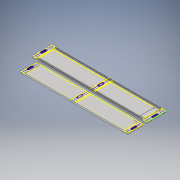
# Autodesk Inventor part: Fixture Base
Saved by Autodesk Inventor 2018 (Build 220112000, 112)
## iProperties
Created: 2016-04-07
Part Number: Fixture Base
Material: Generic
Document SubType Name: Modeling
Designer: Sam Clay
Density: 1 g/cm^3
Appearance: Default
Author: Sam Clay
Autodesk Inventor part; units mm, degrees
ref_plane "YZ Plane" through (0, 0, 0) normal (1, 0, 0) x (0, 1, 0)
ref_plane "XZ Plane" through (0, 0, 0) normal (0, 1, 0) x (-1, 0, 0)
ref_plane "XY Plane" through (0, 0, 0) normal (0, 0, 1) x (1, 0, 0)
sketch "Base Sketch" plane through (0, 0, 0) normal (0, 1, 0) x (-1, 0, 0)
  line L0 (0, 0) -> (1422.4, 0)
  line L1 (1422.4, 0) -> (1422.4, 254)
  line L2 (1320.8, 508) -> (0, 508)
  line L3 (0, 508) -> (0, 304.8)
  line L4 (0, 508) -> (-50.8, 508)
  line L5 (-50.8, 508) -> (-50.8, 304.8)
  line L6 (-50.8, 0) -> (0, 0)
  line L7 (0, 0) -> (0, 254)
  line L8 (1320.8, 508) -> (1371.6, 508)
  line L9 (1371.6, 508) -> (1371.6, 304.8)
  line L10 (1473.2, 0) -> (1422.4, 0)
  line L11 (1422.4, 0) -> (1422.4, 254)
  line L12 (1473.2, 254) -> (1473.2, 0)
  line L13 (0, 254) -> (0, 254)
  line L14 (-50.8, 223.384) -> (-50.8, 0)
  line L15 (1371.6, 304.8) -> (1320.8, 304.8)
  line L16 (1320.8, 304.8) -> (1320.8, 508)
  line L17 (-50.8, 254) -> (-50.8, 223.384)
  line L18 (1422.4, 254) -> (0, 254)
  line L19 (1320.8, 304.8) -> (0, 304.8)
  line L20 (0, 304.8) -> (-50.8, 304.8)
  line L21 (0, 254) -> (-50.8, 254)
  line L22 (0, 304.8) -> (0, 508)
  line L23 (0, 254) -> (0, 0)
  line L24 (1320.8, 304.8) -> (1320.8, 508)
  line L25 (1409.7, 0) -> (1409.7, 254)
  line L26 (12.7, 0) -> (12.7, 254)
  line L27 (1308.1, 304.8) -> (1308.1, 508) construction
  line L28 (12.7, 304.8) -> (12.7, 508) construction
  line L29 (1289.05, 323.85) -> (31.75, 323.85) construction
  line L30 (31.75, 323.85) -> (31.75, 488.95) construction
  line L31 (31.75, 488.95) -> (1289.05, 488.95) construction
  line L32 (1289.05, 488.95) -> (1289.05, 323.85) construction
  line L33 (660.4, 0) -> (660.4, 254)
  line L34 (660.4, 304.8) -> (660.4, 508)
  line L35 (711.2, 0) -> (711.2, 254)
  line L36 (711.2, 304.8) -> (711.2, 508)
  line L37 (647.7, 508) -> (647.7, 304.8)
  line L38 (647.7, 254) -> (647.7, 0)
  line L39 (628.65, 488.95) -> (628.65, 323.85) construction
  line L40 (1473.2, 254) -> (1422.4, 254)
  dimension "d87" = 50.8
  dimension "d88" = 50.8
  dimension "d167" = 203.2
  dimension "d172" = 12.7
  dimension "d173" = 12.7
  dimension "d213" = 12.7
  dimension "d214" = 12.7
  dimension "d215" = 19.05
  dimension "d216" = 19.05
  dimension "d217" = 19.05
  dimension "d218" = 19.05
  dimension "d221" = 660.4
  dimension "d222" = 50.8
  dimension "d230" = 12.7
  dimension "d231" = 19.05
  dimension "d232" = 1524
  dimension "d233" = 50.8
  dimension "d234" = 50.8
  dimension "d235" = 1422.4
  dimension "d236" = 254
  dimension "d237" = 50.8
  constraints: 82 end point, 28 point on line, 23 perpendicular, 22 parallel, 13 coincident, 5 horizontal, 4 midpoint, 1 collinear
  measures "d87" distance of L6.end L6.start
  measures "d88" distance of L10.start L10.end
  measures "d167" distance between parallel lines of L2 L15
  measures "d172" distance between parallel lines of L25 L1
  measures "d173" distance between parallel lines of L23 L26
  measures "d213" distance between parallel lines of L24 L27
  measures "d214" distance between parallel lines of L3 L28
  measures "d215" distance between parallel lines of L29 L19
  measures "d216" distance between parallel lines of L27 L32
  measures "d217" distance between parallel lines of L28 L30
  measures "d218" distance between parallel lines of L2 L31
  measures "d221" distance between parallel lines of L33 L23
  measures "d222" distance between parallel lines of L35 L33
  measures "d230" distance between parallel lines of L37 L34
  measures "d231" distance between parallel lines of L39 L37
  measures "d232" distance between parallel lines of L12 L14
  measures "d233" distance between parallel lines of L9 L16
  measures "d234" distance between parallel lines of L5 L22
  measures "d235" distance between parallel lines of L9 L5
  measures "d236" distance between parallel lines of L18 L0
  measures "d237" distance between parallel lines of L15 L18
extrude "Lower Level" add sketch "Base Sketch" along normal blind 17.78 contours L6 L14 L17 L21 L7 | L1 L40 L12 L10 | L8 L9 L15 L16 | L3 L20 L5 L4
extrude "Base" add sketch "Base Sketch" along normal blind 19.05 contours L7 L18 L26 L0 | L26 L18 L38 L0 | L38 L18 L33 L0 | L33 L18 L35 L0 | L35 L18 L25 L0 | L25 L18 L1 L0 | L16 L19 L36 L2 | L36 L19 L34 L2 | L34 L19 L37 L2 | L37 L19 L3 L2
sketch "Tracks Sketch" plane through (0, 19.05, 0) normal (0, 1, 0) x (1, 0, 0)
  line L0 (-1422.4, 0) -> (-1422.4, -254) projected
  line L1 (0, -254) -> (0, 0) projected
  line L2 (-1422.4, -22.987) -> (0, -22.987)
  line L3 (-1422.4, -3.175) -> (0, -3.175)
  line L4 (-1422.4, -231.013) -> (0, -231.013)
  line L5 (-1422.4, -250.825) -> (0, -250.825)
  line L6 (-63.5, -40.767) -> (-1422.4, -40.767)
  line L7 (-1422.4, -40.767) -> (-1422.4, -231.013)
  line L8 (-63.5, -231.013) -> (-63.5, -40.767)
  circle A0 centre (-67.31, -44.577) radius 8.89
  line L9 (-1371.6, -508) -> (50.8, -508) projected
  line L10 (50.8, -304.8) -> (-1371.6, -304.8) projected
  line L11 (-1473.2, -254) -> (50.8, -254) projected
  line L12 (50.8, 0) -> (-1473.2, 0) projected
  line L13 (-1371.6, -304.8) -> (-1371.6, -508) projected
  line L14 (50.8, -508) -> (50.8, -304.8) projected
  line L15 (-1473.2, 0) -> (-1473.2, -254) projected
  line L16 (50.8, -254) -> (50.8, 0) projected
  point P0 (-660.4, -254)
  point P1 (-1422.4, -223.393)
  point P2 (-1422.4, -254)
  point P3 (-1320.8, -254)
  dimension "d170" = 19.812
  dimension "d171" = 19.812
  dimension "d174" = 63.5
  dimension "d175" = 17.78
  dimension "d178" = 17.78
  dimension "d179" = 5.08
  dimension "d180" = 5.08
  dimension "d219" = 3.175
  dimension "d220" = 3.175
  constraints: 14 end point, 6 point on line, 5 perpendicular, 1 centre point, 1 horizontal, 1 parallel, 6 other
  measures "d170" distance between parallel lines of L5 L4
  measures "d171" distance between parallel lines of L2 L3
  measures "d174" distance between parallel lines of L1 L8
  measures "d175" distance between parallel lines of L2 L6
  measures "d178" diameter of A0
  measures "d179" distance edge to line of A0 L6
  measures "d180" distance edge to line of A0 L8
  measures "d219" distance between parallel lines of L12 L3
  measures "d220" distance between parallel lines of L11 L5
extrude "Pocket side" cut sketch "Tracks Sketch" against normal blind 3.175 contours L6 A0 L8 L4 L0 | A0 L8 L6 | L6 L8 A0
extrude "Tracks" cut sketch "Tracks Sketch" against normal blind 11.43 contours L3 L1 L2 L0 | L4 L1 L5 L0
sketch "Handle Sketch" plane through (0, 17.78, 0) normal (0, 1, 0) x (1, 0, 0)
  line L0 (-1422.4, -40.767) -> (-1422.4, -22.987) projected
  line L1 (-1422.4, -22.987) -> (-1422.4, -3.175) projected
  line L2 (-1422.4, -250.825) -> (-1422.4, -40.767) projected
  line L3 (-1422.4, -254) -> (-1422.4, -250.825) projected
  line L4 (-1422.4, -3.175) -> (-1422.4, 0) projected
  line L5 (-1422.4, 0) -> (-1473.2, 0) projected
  line L6 (-1473.2, 0) -> (-1473.2, -254) projected
  line L7 (50.8, 0) -> (0, 0) projected
  line L8 (0, 0) -> (0, -3.175) projected
  line L9 (0, -3.175) -> (0, -22.987) projected
  line L10 (0, -22.987) -> (0, -231.013) projected
  line L11 (0, -231.013) -> (0, -250.825) projected
  line L12 (0, -250.825) -> (0, -254) projected
  line L13 (0, -254) -> (50.8, -254) projected
  line L14 (50.8, -254) -> (50.8, 0) projected
  line L15 (0, -508) -> (50.8, -508) projected
  line L16 (50.8, -508) -> (50.8, -304.8) projected
  line L17 (50.8, -304.8) -> (0, -304.8) projected
  line L18 (0, -304.8) -> (0, -508) projected
  line L19 (-1320.8, -508) -> (-1320.8, -304.8) projected
  line L20 (-1320.8, -304.8) -> (-1371.6, -304.8) projected
  line L21 (-1371.6, -304.8) -> (-1371.6, -508) projected
  line L22 (-1371.6, -508) -> (-1320.8, -508) projected
  line L23 (-1422.4, 0) -> (-1473.2, 0) construction
  line L24 (31.75, 0) -> (31.75, -508) construction
  line L25 (-1454.15, -88.9) -> (-1454.15, -165.1) construction
  line L26 (-1466.85, -101.6) -> (-1466.85, -152.4)
  line L27 (-1441.45, -152.4) -> (-1441.45, -101.6)
  arc A0 (-1441.45, -101.6) -> (-1466.85, -101.6) centre (-1454.15, -101.6) ccw
  arc A1 (-1466.85, -152.4) -> (-1441.45, -152.4) centre (-1454.15, -152.4) ccw
  line L28 (31.75, -88.9) -> (31.75, -165.1) construction
  line L29 (19.05, -101.6) -> (19.05, -152.4)
  line L30 (44.45, -152.4) -> (44.45, -101.6)
  arc A2 (44.45, -101.6) -> (19.05, -101.6) centre (31.75, -101.6) ccw
  arc A3 (19.05, -152.4) -> (44.45, -152.4) centre (31.75, -152.4) ccw
  line L31 (-1352.55, -368.3) -> (-1352.55, -444.5) construction
  line L32 (-1365.25, -381) -> (-1365.25, -431.8)
  line L33 (-1339.85, -431.8) -> (-1339.85, -381)
  arc A4 (-1339.85, -381) -> (-1365.25, -381) centre (-1352.55, -381) ccw
  arc A5 (-1365.25, -431.8) -> (-1339.85, -431.8) centre (-1352.55, -431.8) ccw
  line L34 (31.75, -368.3) -> (31.75, -444.5) construction
  line L35 (19.05, -381) -> (19.05, -431.8)
  line L36 (44.45, -431.8) -> (44.45, -381)
  arc A6 (44.45, -381) -> (19.05, -381) centre (31.75, -381) ccw
  arc A7 (19.05, -431.8) -> (44.45, -431.8) centre (31.75, -431.8) ccw
  arc A8 (-679.45, -381) -> (-704.85, -381) centre (-692.15, -381) ccw
  line L37 (-704.85, -381) -> (-704.85, -431.8)
  line L38 (-679.45, -431.8) -> (-679.45, -381)
  arc A9 (-704.85, -431.8) -> (-679.45, -431.8) centre (-692.15, -431.8) ccw
  arc A10 (-704.85, -152.4) -> (-679.45, -152.4) centre (-692.15, -152.4) ccw
  line L39 (-704.85, -101.6) -> (-704.85, -152.4)
  arc A11 (-679.45, -101.6) -> (-704.85, -101.6) centre (-692.15, -101.6) ccw
  line L40 (-679.45, -152.4) -> (-679.45, -101.6)
  line L41 (-1473.2, -254) -> (-1422.4, -254) projected
  line L42 (-1454.15, 0) -> (-1454.15, -254) construction
  line L43 (-1473.2, -254) -> (-1422.4, -254) construction
  line L44 (-1320.8, -304.8) -> (-1371.6, -304.8) construction
  line L45 (-1352.55, -304.8) -> (-1352.55, -508) construction
  line L46 (-1371.6, -508) -> (-1320.8, -508) construction
  point P0 (-1454.15, -25.4)
  point P1 (-1454.15, -50.8)
  point P2 (-1454.15, -203.2)
  point P3 (-1454.15, -228.6)
  point P4 (-1352.55, -317.5)
  point P5 (-1352.55, -342.9)
  point P6 (-1352.55, -469.9)
  point P7 (-1352.55, -495.3)
  point P8 (31.75, -495.3)
  point P9 (31.75, -469.9)
  point P10 (31.75, -342.9)
  point P11 (31.75, -317.5)
  point P12 (31.75, -228.6)
  point P13 (31.75, -203.2)
  point P14 (31.75, -50.8)
  point P15 (31.75, -25.4)
  point P16 (-1454.15, -127)
  point P17 (31.75, -127)
  point P18 (-1352.55, -406.4)
  point P19 (31.75, -406.4)
  point P20 (-692.15, -25.4)
  point P21 (-692.15, -50.8)
  point P22 (-692.15, -203.2)
  point P23 (-692.15, -228.6)
  point P24 (-692.15, -317.5)
  point P25 (-692.15, -342.9)
  point P26 (-692.15, -469.9)
  point P27 (-692.15, -495.3)
  dimension "d182" = 19.05
  dimension "d183" = 25.4
  dimension "d184" = 25.4
  dimension "d186" = 25.4
  dimension "d187" = 25.4
  dimension "d188" = 25.4
  dimension "d189" = 25.4
  dimension "d190" = 25.4
  dimension "d191" = 12.7
  dimension "d192" = 25.4
  dimension "d193" = 12.7
  dimension "d194" = 25.4
  dimension "d195" = 12.7
  dimension "d196" = 25.4
  dimension "d197" = 12.7
  dimension "d198" = 25.4
  dimension "d199" = 76.2
  dimension "d200" = 25.4
  dimension "d201" = 127
  dimension "d202" = 76.2
  dimension "d203" = 25.4
  dimension "d204" = 127
  dimension "d205" = 76.2
  dimension "d206" = 25.4
  dimension "d207" = 76.2
  dimension "d208" = 25.4
  dimension "d209" = 101.6
  dimension "d210" = 101.6
  dimension "d225" = 723.9
  dimension "d238" = 19.05
  dimension "d239" = 25.4
  dimension "d240" = 19.05
  constraints: 44 end point, 32 point on circle, 25 point on line, 16 tangent, 12 centre point, 5 midpoint, 4 parallel, 2 horizontal, 2 perpendicular, 43 other
  measures "d183" distance from line of point (-1454.15, -25.4) L5
  measures "d184" distance of point (-1454.15, -25.4) point (-1454.15, -50.8)
  measures "d186" distance of point (-1454.15, -203.2) point (-1454.15, -228.6)
  measures "d187" distance from line of point (31.75, -25.4) L7
  measures "d188" distance of point (31.75, -50.8) point (31.75, -25.4)
  measures "d189" distance from line of L13 point (31.75, -228.6)
  measures "d190" distance of point (31.75, -203.2) point (31.75, -228.6)
  measures "d191" distance from line of point (-1352.55, -317.5) L20
  measures "d192" distance of point (-1352.55, -342.9) point (-1352.55, -317.5)
  measures "d193" distance from line of L22 point (-1352.55, -495.3)
  measures "d194" distance of point (-1352.55, -469.9) point (-1352.55, -495.3)
  measures "d195" distance from line of L15 point (31.75, -495.3)
  measures "d196" distance of point (31.75, -469.9) point (31.75, -495.3)
  measures "d197" distance from line of point (31.75, -317.5) L17
  measures "d198" distance of point (31.75, -342.9) point (31.75, -317.5)
  measures "d199" distance of L25.start L25.end
  measures "d200" diameter of A1
  measures "d201" distance from line of L5 point (-1454.15, -127)
  measures "d202" distance of L28.start L28.end
  measures "d203" diameter of A3
  measures "d204" distance from line of L7 point (31.75, -127)
  measures "d205" distance of L31.start L31.end
  measures "d206" diameter of A5
  measures "d207" distance of L34.start L34.end
  measures "d208" diameter of A7
  measures "d209" distance from line of point (-1352.55, -406.4) L20
  measures "d210" distance from line of point (31.75, -406.4) L17
  measures "d225" distance of point (31.75, -25.4) point (-692.15, -25.4)
  measures "d238" distance between parallel lines of L42 L6
  measures "d239" distance of L42.end point (-1454.15, -228.6)
  measures "d240" distance between parallel lines of L45 L21
sketch "Origin Sketch" plane through (0, 19.05, 0) normal (0, 1, 0) x (1, 0, 0)
  line L0 (50.8, -254) -> (50.8, 0)
  line L1 (-1422.4, -40.767) -> (-75.3422, -40.767) projected
  line L2 (-12.7, 0) -> (-12.7, -254) projected
  line L3 (0, -304.8) -> (-1320.8, -304.8) projected
  line L4 (0, -304.8) -> (0, -508) projected
  line L5 (-647.7, -508) -> (-647.7, -304.8) projected
  line L6 (-660.4, -304.8) -> (-660.4, -508) projected
  line L7 (-711.2, -304.8) -> (-711.2, -508) projected
  line L8 (-647.7, -254) -> (-647.7, 0) projected
  line L9 (-660.4, 0) -> (-660.4, -254) projected
  line L10 (-711.2, 0) -> (-711.2, -254) projected
  line L11 (-12.7, -304.8) -> (-12.7, -508) construction
  line L12 (-628.65, -488.95) -> (-628.65, -323.85) construction
  line L13 (-1289.05, -323.85) -> (-31.75, -323.85) construction
  line L14 (-31.75, -488.95) -> (-1289.05, -488.95) construction
  line L15 (-31.75, -323.85) -> (-31.75, -488.95) construction
  line L16 (-1289.05, -488.95) -> (-1289.05, -323.85) construction
  line L17 (-1308.1, -304.8) -> (-1308.1, -508) construction
  line L18 (-1409.7, 0) -> (-1409.7, -254) projected
  point P0 (0, 0)
  point P1 (-12.7, -40.767)
  point P2 (-711.2, -508)
  point P3 (50.8, -508)
  point P4 (-25.4, -317.5)
  dimension "d211" = 12.7
  dimension "d212" = 25.4
  constraints: 2 end point, 2 point on line
  measures "d211" distance from line of L3 point (-25.4, -317.5)
  measures "d212" distance from line of L4 point (-25.4, -317.5)
extrude "Handles" cut sketch "Handle Sketch" along normal through all both and the other way through all contours A0 L27 A1 L26 | A2 L30 A3 L29 | A4 L33 A5 L32 | A6 L36 A7 L35
body "Solid1"
